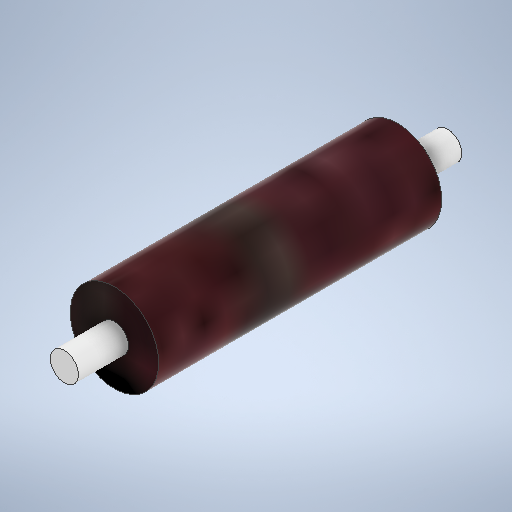
# Autodesk Inventor part: Conveyor_002_001
Saved by Autodesk Inventor 2026 (Build 300175000, 175)
## iProperties
Created: 2025-05-22
Part Number: Conveyor_002_001
Material: ABS Plastic
Document SubType Name: Modeling
Designer: carlo
Density: 1.06 g/cm^3
Appearance: Smooth - White
Author: carlo
Autodesk Inventor part; units mm, degrees
ref_plane "YZ Plane" through (0, 0, 0) normal (1, 0, 0) x (0, 1, 0)
ref_plane "XZ Plane" through (0, 0, 0) normal (0, 1, 0) x (-1, 0, 0)
ref_plane "XY Plane" through (0, 0, 0) normal (0, 0, 1) x (1, 0, 0)
sketch "Sketch1" plane through (0, 0, 0) normal (0, 0, 1) x (1, 0, 0)
  circle A0 centre (0, 0) radius 7.5
  circle A1 centre (0, 0) radius 2.4
  dimension "d0" = 15
  dimension "d1" = 4.8
  constraints: 2 centre point, 2 coincident
  measures "d0" diameter of A0
  measures "d1" diameter of A1
extrude "Extrusion1" add sketch "Sketch1" along normal mid plane 65 contours A1
extrude "Extrusion2" add sketch "Sketch1" along normal mid plane 48
body "Solid1"
